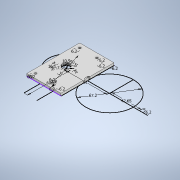
# Autodesk Inventor part: motor mount layer
Saved by Autodesk Inventor 2022 (Build 260153000, 153)
## iProperties
Created: 2021-11-30
Part Number: motor mount layer
Material: Generic
Document SubType Name: Modeling
Designer: a-dubs
Density: 1 g/cm^3
Appearance: Default
Author: a-dubs
Autodesk Inventor part; units mm, degrees
ref_plane "YZ Plane" through (0, 0, 0) normal (1, 0, 0) x (0, 1, 0)
ref_plane "XZ Plane" through (0, 0, 0) normal (0, 1, 0) x (-1, 0, 0)
ref_plane "XY Plane" through (0, 0, 0) normal (0, 0, 1) x (1, 0, 0)
sketch "Sketch1" plane through (0, 0, 0) normal (0, 1, 0) x (-1, 0, 0)
  line L0 (0, 0) -> (61, 0)
  circle A0 centre (0, 0) radius 33.6
  circle A1 centre (61, 0) radius 8.05
  line L1 (69.05, 0) -> (69.05, 7.5)
  line L2 (69.05, 7.5) -> (69.05, -7.5)
  line L3 (69.05, -7.5) -> (63.9245, -7.5)
  line L4 (69.05, 7.5) -> (63.9245, 7.5)
  line L5 (69.05, 7.5) -> (72.05, 7.5)
  line L6 (72.05, 7.5) -> (72.05, -7.5)
  line L7 (72.05, -7.5) -> (69.05, -7.5)
  line L8 (52.95, 0) -> (47.95, 0)
  line L9 (61, 8.05) -> (61, 13.05)
  line L10 (72.05, 0) -> (77.05, 0)
  line L11 (61, -8.05) -> (61, -13.05)
  line L12 (47.95, 13.05) -> (77.05, 13.05)
  line L13 (77.05, 13.05) -> (77.05, -13.05)
  line L14 (77.05, -13.05) -> (47.95, -13.05)
  line L15 (47.95, -13.05) -> (47.95, 13.05)
  line L16 (72.05, 7.5) -> (72.05, 10.5)
  line L17 (72.05, 10.5) -> (63.9245, 10.5)
  line L18 (63.9245, 10.5) -> (63.9245, 7.5)
  line L19 (72.05, -7.5) -> (72.05, -10.5)
  line L20 (72.05, -10.5) -> (63.9245, -10.5)
  line L21 (63.9245, -10.5) -> (63.9245, -7.5)
  line L22 (61, 0) -> (61, 60)
  line L23 (0, 0) -> (-42.65, 0)
  line L24 (-42.65, 0) -> (-47.65, 0)
  line L25 (-47.65, 0) -> (-53.85, 0)
  line L26 (0, 0) -> (0, -33.6)
  line L27 (0, 0) -> (42.65, 0)
  line L28 (42.65, 0) -> (42.65, 60)
  line L29 (42.65, 0) -> (42.65, -33.6)
  circle A2 centre (61, 0) radius 25
  line L30 (42.65, 25) -> (42.65, 31.2)
  line L31 (42.65, 31.2) -> (48.85, 31.2)
  line L32 (42.65, -25) -> (42.65, -31.2)
  line L33 (42.65, -31.2) -> (48.85, -31.2)
  circle A3 centre (48.85, 31.2) radius 3.1
  circle A4 centre (48.85, 31.2) radius 1.6
  circle A5 centre (48.85, 31.2) radius 1.45
  circle A6 centre (48.85, -31.2) radius 3.1
  circle A7 centre (48.85, -31.2) radius 1.6
  circle A8 centre (48.85, -31.2) radius 1.45
  circle A9 centre (73.15, 31.2) radius 3.1
  circle A10 centre (73.15, 31.2) radius 1.6
  circle A11 centre (73.15, 31.2) radius 1.45
  circle A12 centre (73.15, -31.2) radius 3.1
  circle A13 centre (73.15, -31.2) radius 1.45
  circle A14 centre (73.15, -31.2) radius 1.6
  line L34 (73.15, 31.2) -> (79.35, 31.2)
  line L35 (73.15, -31.2) -> (79.35, -31.2)
  line L36 (36, 0) -> (31, 0)
  line L37 (31, 0) -> (31, -31.2)
  line L38 (31, -31.2) -> (31, -37.4)
  line L39 (31, -37.4) -> (79.35, -37.4)
  line L40 (79.35, -37.4) -> (79.35, 31.2)
  line L41 (79.35, 31.2) -> (79.35, 37.4)
  line L42 (79.35, 37.4) -> (31, 37.4)
  line L43 (31, 37.4) -> (31, 0)
  line L44 (42.65, -33.6) -> (42.65, -37.4)
  circle A15 centre (61, 0) radius 5.25
  point P0 (42.65, 37.4)
  dimension "d1" = 67.2
  dimension "d16" = 50
  dimension "d0" = 61
  dimension "d2" = 16.1
  dimension "d3" = 7.5
  dimension "d4" = 15
  dimension "d5" = 3
  dimension "d6" = 5
  dimension "d7" = 5
  dimension "d8" = 5
  dimension "d9" = 5
  dimension "d10" = 3
  dimension "d11" = 60
  dimension "d13" = 42.65
  dimension "d14" = 5
  dimension "d15" = 6.2
  dimension "d17" = 6.2
  dimension "d18" = 6.2
  dimension "d19" = 6.2
  dimension "d20" = 6.2
  dimension "d21" = 6.2
  dimension "d22" = 3.2
  dimension "d23" = 2.9
  dimension "d24" = 6.2
  dimension "d25" = 6.2
  dimension "d26" = 5
  dimension "d27" = 6.2
  dimension "d28" = 6.2
  dimension "d31" = 10.5
  constraints: 90 end point, 14 centre point, 14 coincident, 14 perpendicular, 13 point on line, 12 symmetric about line, 9 vertical, 8 horizontal, 6 point on circle, 3 parallel, 1 horizontal alignment, 1 midpoint, 1 vertical alignment, 13 other
  measures "d0" distance of L0.start L0.end
  measures "d2" diameter of A1
  measures "d3" distance of L1.start L1.end
  measures "d4" distance of L1.end L2.end
  measures "d5" distance of L1.end L5.end
  measures "d6" distance of L8.start L8.end
  measures "d7" distance of L9.start L9.end
  measures "d8" distance of L10.start L10.end
  measures "d9" distance of L11.start L11.end
  measures "d10" distance of L5.end L16.end
  measures "d11" distance of L22.start L22.end
  measures "d13" distance of L23.start L23.end
  measures "d14" distance of L23.end L24.end
  measures "d15" distance of L24.end L25.end
  measures "d17" distance of L30.start L30.end
  measures "d18" distance of L30.end L31.end
  measures "d19" distance of L32.start L32.end
  measures "d20" distance of L32.end L33.end
  measures "d21" diameter of A3
  measures "d22" diameter of A4
  measures "d23" diameter of A5
  measures "d24" distance of L34.start L34.end
  measures "d25" distance of L35.start L35.end
  measures "d26" distance of L36.start L36.end
  measures "d27" distance of L37.end L38.end
  measures "d28" distance of L34.end L41.end
  measures "d31" diameter of A15
extrude "Extrusion1" add sketch "Sketch1" along normal blind 3.2 contours L43 A0 L0 | L0 A0 L37 | A0 L43 L42 L28 A2 L0 | L0 A2 L29 L44 L39 L38 L37 A0 | A2 L28 L0 | L0 L29 A2 | L28 A2 L22 L12 L15 L0 | L0 L15 L14 L13 L12 L22 A2 L40 L29 | L28 L42 L22 A2 | A2 L40 L39 L44 L29 | L15 L12 L9 A1 L0 | L0 A1 L11 L14 L15 | L22 L42 L41 L40 A2 | A1 L22 A15 L0 | L0 A15 L22 A1 | L12 L13 L10 L6 L16 L17 L18 A1 L9 | A1 L21 L20 L19 L6 L10 L13 L14 L11 | L4 L1 A1 | L18 L17 L16 L5 L4 | A1 L2 L3 | L3 L7 L19 L20 L21 | L1 L5 L6 L7 L2 | A3 | A6 | A9 | A12
body "Solid1"
